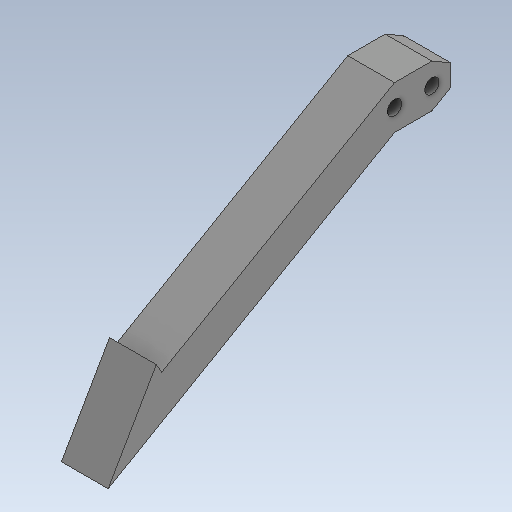
# Autodesk Inventor part: HexFlipperSpike
Saved by Autodesk Inventor 2020 (Build 240168000, 168)
## iProperties
Created: 2023-12-22
Part Number: HexFlipperSpike
Material: H TPU
Document SubType Name: Modeling
Designer: smz3rm
Density: 0.941117 g/cm^3
Appearance: Generic(1)
Mass: 5.83903 g
Surface Area: 32.4675 cm^2
Volume: 6.20436 cm^3
FlipperSpikeReach: 60.308 mm
FlipperSpikeTipAngle: 60.00 deg
FlipperSpikeTipOffset: 2.000 mm
Author: smz3rm
Autodesk Inventor part; units mm, degrees
ref_plane "YZ Plane" through (0, 0, 0) normal (1, 0, 0) x (0, 1, 0)
ref_plane "XZ Plane" through (0, 0, 0) normal (0, 1, 0) x (-1, 0, 0)
ref_plane "XY Plane" through (0, 0, 0) normal (0, 0, 1) x (1, 0, 0)
sketch "Sketch1" plane through (0, 0, 0) normal (1, 0, 0) x (0, 1, 0)
  line L0 (2.3094, 8) -> (-2.3094, 8)
  line L1 (-2.3094, 8) -> (-2.3094, -8)
  line L2 (-2.3094, -8) -> (2.3094, -8)
  line L3 (2.3094, -8) -> (2.3094, 8)
  line L4 (2.3094, 8) -> (-2.3094, -8) construction
  line L5 (-2.3094, 8) -> (2.3094, -8) construction
  line L6 (2.3094, 8) -> (-24.153, 53.8342)
  line L7 (2.3094, -8) -> (-2.3094, -8)
  line L8 (-2.3094, -8) -> (-4.6188, -4)
  line L9 (-4.6188, -4) -> (-2.3094, 0)
  line L10 (-2.3094, 0) -> (2.3094, 0)
  line L11 (2.3094, 0) -> (4.6188, -4)
  line L12 (4.6188, -4) -> (2.3094, -8)
  line L13 (0, -22.6597) -> (0, 79.958) projected
  line L14 (2.3094, 8) -> (4.6188, 4)
  line L15 (4.6188, 4) -> (2.3094, 0)
  line L16 (2.3094, 0) -> (-2.3094, 0)
  line L17 (-2.3094, 0) -> (-4.6188, 4)
  line L18 (-4.6188, 4) -> (-2.3094, 8)
  line L19 (-2.3094, 8) -> (2.3094, 8)
  line L20 (4.6188, 4) -> (4.6188, -4)
  line L21 (-4.6188, 4) -> (-4.6188, -4)
  circle A0 centre (0, -4) radius 1.55
  circle A1 centre (0, 4) radius 1.55
  line L22 (2.3094, 8) -> (2.3094, 5.0078)
  line L23 (-40.0094, 65.2983) -> (-22.153, 54.9889)
  line L24 (-22.153, 54.9889) -> (-24.153, 53.8342)
  line L25 (-4.6188, 4) -> (-40.0094, 65.2983)
  point P0 (0, 0)
  point P1 (2.3094, 8)
  point P2 (-3.4641, 6)
  point P3 (0, 8)
  point P4 (0, 12)
  dimension "d3" = 4.6188
  dimension "d4" = 16
  dimension "d15" = 8
  dimension "d16" = 8
  dimension "d18" = 3.1
  dimension "d19" = 3.1
  dimension "d20" = 4.6188
  dimension "d23" = 2
  dimension "d24" = 40.0094
  dimension "d25" = 60
  dimension "d26" = 30
  dimension "d27" = 73.2983
  constraints: 52 end point, 3 collinear, 3 midpoint, 3 parallel, 2 centre point, 2 horizontal, 2 perpendicular, 2 point on line, 2 vertical, 1 coincident, 26 other
  measures "d3" distance of L2.end L1.end
  measures "d4" distance of L0.end L1.end
  measures "d15" distance between parallel lines of L8 L11
  measures "d16" distance between parallel lines of L17 L14
  measures "d18" diameter of A0
  measures "d19" diameter of A1
  measures "d20" distance of L7.end L7.start
  measures "d23" horizontal distance of L23.end L6.end
  measures "d24" horizontal distance of L23.start A1.centre
  measures "d25" angle of L13 L23
  measures "d26" angle of L13 L6
  measures "d27" vertical distance of L23.start L2.end
extrude "Extrusion2" add sketch "Sketch1" along normal blind 10 contours L3 L10 L13 A1 L0 | L14 L15 L3 | L0 L13 L6 | L13 A1 L10 L1 L0 | L0 L18 L25 L23 L24 L6 L13 | L20 L11 L15 | L1 L17 L18 | L11 L12 L3 | L3 L2 L13 A0 L10 | L10 L13 A0 L2 L1 | L1 L8 L9 | L9 L21 L17
equation "\"d3\" = FlipperArmThickness"
equation "\"d4\" = 2 * M3ScrewInsertBrim"
equation "\"d15\" = M3ScrewInsertBrim"
equation "\"d16\" = M3ScrewInsertBrim"
equation "\"d18\" = M3ScrewDia"
equation "\"d19\" = M3ScrewDia"
equation "\"d23\" = FlipperSpikeTipOffset"
equation "\"d24\" = FlipperSpikeDrop"
equation "\"d25\" = FlipperSpikeTipAngle"
equation "\"d26\" = FlipperSpikeAngle"
equation "\"d32\" = FlipperSpikeWidth"
equation "\"FlipperSpikeReach\" = d27 - 0.433013 * BodyHeight"
equation "\"FlipperSpikeTipAngle\" = 60deg"
equation "\"FlipperSpikeTipOffset\" = 2"
equation "\"FlipperArmThickness\" = 4.618802"
equation "\"M3ScrewInsertBrim\" = 8"
equation "\"M3ScrewDia\" = 3.1"
equation "\"FlipperSpikeDrop\" = 40.009401"
equation "\"FlipperSpikeAngle\" = 30deg"
equation "\"FlipperSpikeWidth\" = 10"
equation "\"BodyHeight\" = 30"
body "Solid2"
